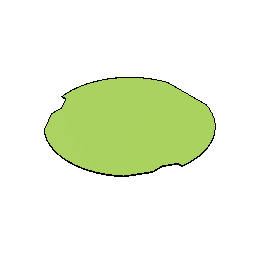
bed_shape (Autodesk Fusion 360 design; units mm, degrees)
Autodesk Fusion 360 part; units mm, degrees
sketch "Sketch1" plane through (0, 0, 0) normal (0, 0, 1) x (1, 0, 0)
  circle A0 centre (0, 0) radius 95
  line L0 (0, 0) -> (120, 0) construction
  line L1 (0, 0) -> (103.923, -60) construction
  line L2 (0, 0) -> (120, 0) construction
  line L3 (30.4138, 90) -> (-30.4138, 90)
  line L4 (62.7354, -71.3391) -> (93.1492, -18.6609)
  line L5 (0, -100) -> (0, 100) construction
  line L6 (78.923, -12) -> (103.923, -12)
  line L7 (103.923, -12) -> (103.923, -60) construction
  line L8 (103.923, -60) -> (78.923, -60) construction
  line L9 (78.923, -60) -> (78.923, -12)
  circle A1 centre (0, 0) radius 120 construction
  line L10 (78.923, -27.3013) -> (87.7572, -12)
  line L11 (-78.923, -27.3013) -> (-87.7572, -12)
  line L12 (-62.7354, -71.3391) -> (-93.1492, -18.6609)
  line L13 (-78.923, -60) -> (-78.923, -12)
  line L14 (-78.923, -12) -> (-103.923, -12)
  dimension "d1" = 190
  dimension "d5" = 30
  dimension "d14" = 90
  dimension "d15" = 90
  dimension "d18" = 240
  dimension "d19" = 25
  dimension "d20" = 48
  dimension "d22" = 8
  dimension "d24" = 12
  dimension "d25" = 78.923
  dimension "d26" = 83.5117
  constraint coincident A0.centre L0.start
  constraint horizontal L0
  constraint horizontal L2
  constraint horizontal L3
  constraint coincident A0 L4.start
  constraint coincident A0 L4.end
  constraint perpendicular L1 L4
  constraint vertical L5
  constraint coincident A0 L3.end
  constraint coincident A0 L3.start
  constraint horizontal L6
  constraint vertical L7
  constraint horizontal L8
  constraint vertical L9
  constraint concentric A0 A1
  constraint coincident L1.end A1
  constraint parallel L4 L10
  constraint coincident L6 L10.end
  constraint coincident L9 L10.start
  constraint symmetric L4.start L5 L12.start
  constraint symmetric L4.end L5 L12.end
  constraint symmetric L5 L6.start L13.end
  constraint symmetric L5 L6.end L14.end
  constraint symmetric L5 L8.end L13.start
  constraint symmetric L5 L10.end L11.end
  constraint symmetric L5 L10.start L11.start
  measures "d1" diameter of A0
  measures "d5" angle of L1 L2
  measures "d14" distance of A0.centre L3
  measures "d15" distance of A0.centre L4
  measures "d18" diameter of A1
  measures "d19" distance of L1.end L8.end
  measures "d20" distance of L1.end L6.end
  measures "d22" distance of L4 L10
  measures "d24" distance of L2 L6
  measures "d25" distance of L9 A0.centre
  measures "d26" distance of A0.centre L11.start
extrude "Extrude1" add sketch "Sketch1" along normal blind 1 contours A0 L3 L4 L6 L9 L12 L13 L14 | L6 L9 L10 | L11 L13 L14
